Autodesk Inventor part; units mm, degrees
(part 2 of 2)
  spline S240 degree 2 poles (-24.576, 3.7543) (-24.576, 3.8655) (-24.644, 4.0034) (-24.7057, 4.0425) knots 0 0 0 1 2 2 2
  spline S241 degree 2 poles (-24.7057, 4.0425) (-24.7675, 4.0816) (-24.9445, 4.1063) (-25.0392, 4.1063) knots 0 0 0 1 2 2 2
  spline S242 degree 2 poles (-25.0392, 4.1063) (-25.1503, 4.1063) (-25.4508, 4.0404) (-25.6011, 3.9766) knots 0 0 0 1 2 2 2
  line L294 (-25.6011, 3.9766) -> (-25.6196, 3.9766)
  line L295 (-25.6196, 3.9766) -> (-25.6196, 4.3039)
  spline S243 degree 2 poles (-25.6196, 4.3039) (-25.5311, 4.3286) (-25.1997, 4.3903) (-25.0371, 4.3903) knots 0 0 0 1 2 2 2
  spline S244 degree 2 poles (-25.0371, 4.3903) (-24.8395, 4.3903) (-24.5699, 4.3286) (-24.4628, 4.2483) knots 0 0 0 1 2 2 2
  spline S245 degree 2 poles (-24.4628, 4.2483) (-24.3578, 4.1701) (-24.2549, 3.921) (-24.2549, 3.742) knots 0 0 0 1 2 2 2
  line L296 (-24.2549, 3.742) -> (-24.2549, 2.439)
  line L297 (-24.2549, 2.439) -> (-24.576, 2.439)
  line L298 (-24.576, 2.439) -> (-24.576, 2.6407)
  line L299 (-24.576, 2.9083) -> (-24.576, 3.4373)
  spline S246 degree 2 poles (-24.576, 3.4373) (-24.6913, 3.427) (-25.0392, 3.392) (-25.1482, 3.3591) knots 0 0 0 1 2 2 2
  spline S247 degree 2 poles (-25.1482, 3.3591) (-25.2759, 3.32) (-25.4426, 3.1574) (-25.4426, 3.0133) knots 0 0 0 1 2 2 2
  spline S248 degree 2 poles (-25.4426, 3.0133) (-25.4426, 2.8486) (-25.2573, 2.6819) (-25.0803, 2.6819) knots 0 0 0 1 2 2 2
  spline S249 degree 2 poles (-25.0803, 2.6819) (-24.9301, 2.6819) (-24.6831, 2.8116) (-24.576, 2.9083) knots 0 0 0 1 2 2 2
  line L300 (-20.836, 2.439) -> (-21.2744, 2.439)
  line L301 (-21.2744, 2.439) -> (-22.2028, 3.6205)
  line L302 (-22.2028, 3.6205) -> (-22.351, 3.4538)
  line L303 (-22.351, 3.4538) -> (-22.351, 2.439)
  line L304 (-22.351, 2.439) -> (-22.6885, 2.439)
  line L305 (-22.6885, 2.439) -> (-22.6885, 4.979)
  line L306 (-22.6885, 4.979) -> (-22.351, 4.979)
  line L307 (-22.351, 4.979) -> (-22.351, 3.8119)
  line L308 (-22.351, 3.8119) -> (-21.3094, 4.979)
  line L309 (-21.3094, 4.979) -> (-20.8978, 4.979)
  line L310 (-20.8978, 4.979) -> (-21.9496, 3.8449)
  line L311 (-21.9496, 3.8449) -> (-20.836, 2.439)
  line L312 (-19.6483, 4.0013) -> (-19.6648, 4.0013)
  spline S250 degree 2 poles (-19.6648, 4.0013) (-19.7019, 4.0116) (-19.7821, 4.0157) (-19.8377, 4.0157) knots 0 0 0 1 2 2 2
  spline S251 degree 2 poles (-19.8377, 4.0157) (-19.9674, 4.0157) (-20.2226, 3.9025) (-20.3379, 3.7914) knots 0 0 0 1 2 2 2
  line L313 (-20.3379, 3.7914) -> (-20.3379, 2.439)
  line L314 (-20.3379, 2.439) -> (-20.659, 2.439)
  line L315 (-20.659, 2.439) -> (-20.659, 4.3451)
  line L316 (-20.659, 4.3451) -> (-20.3379, 4.3451)
  line L317 (-20.3379, 4.3451) -> (-20.3379, 4.061)
  spline S252 degree 2 poles (-20.3379, 4.061) (-20.1629, 4.2174) (-19.9015, 4.3451) (-19.778, 4.3451) knots 0 0 0 1 2 2 2
  spline S253 degree 2 poles (-19.778, 4.3451) (-19.7286, 4.3451) (-19.6792, 4.3409) (-19.6483, 4.3348) knots 0 0 0 1 2 2 2
  line L318 (-19.6483, 4.3348) -> (-19.6483, 4.0013)
  line L319 (-19.6339, 5.2981) -> (-20.023, 4.6517)
  line L320 (-20.023, 4.6517) -> (-20.4099, 4.6517)
  line L321 (-20.4099, 4.6517) -> (-20.799, 5.2981)
  line L322 (-20.799, 5.2981) -> (-20.5273, 5.2981)
  line L323 (-20.5273, 5.2981) -> (-20.2123, 4.8617)
  line L324 (-20.2123, 4.8617) -> (-19.8974, 5.2981)
  line L325 (-19.8974, 5.2981) -> (-19.6339, 5.2981)
  line L326 (-19.072, 2.439) -> (-19.3931, 2.439)
  line L327 (-19.3931, 2.439) -> (-19.3931, 4.3451)
  line L328 (-19.3931, 4.3451) -> (-19.072, 4.3451)
  line L329 (-19.072, 4.3451) -> (-19.072, 2.439)
  line L330 (-19.0494, 4.662) -> (-19.4137, 4.662)
  line L331 (-19.4137, 4.662) -> (-19.4137, 4.9955)
  line L332 (-19.4137, 4.9955) -> (-19.0494, 4.9955)
  line L333 (-19.0494, 4.9955) -> (-19.0494, 4.662)
  line L334 (-17.3492, 2.439) -> (-18.7488, 2.439)
  line L335 (-18.7488, 2.439) -> (-18.7488, 2.6778)
  line L336 (-18.7488, 2.6778) -> (-17.7526, 4.0816)
  line L337 (-17.7526, 4.0816) -> (-18.7077, 4.0816)
  line L338 (-18.7077, 4.0816) -> (-18.7077, 4.3451)
  line L339 (-18.7077, 4.3451) -> (-17.3677, 4.3451)
  line L340 (-17.3677, 4.3451) -> (-17.3677, 4.1166)
  line L341 (-17.3677, 4.1166) -> (-18.3681, 2.7087)
  line L342 (-18.3681, 2.7087) -> (-17.3492, 2.7087)
  line L343 (-17.3492, 2.7087) -> (-17.3492, 2.439)
  line L344 (-17.4665, 5.2981) -> (-17.8555, 4.6517)
  line L345 (-17.8555, 4.6517) -> (-18.2425, 4.6517)
  line L346 (-18.2425, 4.6517) -> (-18.6315, 5.2981)
  line L347 (-18.6315, 5.2981) -> (-18.3598, 5.2981)
  line L348 (-18.3598, 5.2981) -> (-18.0449, 4.8617)
  line L349 (-18.0449, 4.8617) -> (-17.73, 5.2981)
  line L350 (-17.73, 5.2981) -> (-17.4665, 5.2981)
  line L351 (-16.7214, 2.439) -> (-17.0425, 2.439)
  line L352 (-17.0425, 2.439) -> (-17.0425, 4.3451)
  line L353 (-17.0425, 4.3451) -> (-16.7214, 4.3451)
  line L354 (-16.7214, 4.3451) -> (-16.7214, 2.439)
  line L355 (-16.355, 5.2981) -> (-16.8202, 4.66)
  line L356 (-16.8202, 4.66) -> (-17.0754, 4.66)
  line L357 (-17.0754, 4.66) -> (-16.7708, 5.2981)
  line L358 (-16.7708, 5.2981) -> (-16.355, 5.2981)
  line L359 (-14.6713, 2.439) -> (-15.0932, 2.439)
  line L360 (-15.0932, 2.439) -> (-15.8013, 3.3591)
  line L361 (-15.8013, 3.3591) -> (-15.9289, 3.2356)
  line L362 (-15.9289, 3.2356) -> (-15.9289, 2.439)
  line L363 (-15.9289, 2.439) -> (-16.25, 2.439)
  line L364 (-16.25, 2.439) -> (-16.25, 5.0922)
  line L365 (-16.25, 5.0922) -> (-15.9289, 5.0922)
  line L366 (-15.9289, 5.0922) -> (-15.9289, 3.5402)
  line L367 (-15.9289, 3.5402) -> (-15.1756, 4.3451)
  line L368 (-15.1756, 4.3451) -> (-14.7762, 4.3451)
  line L369 (-14.7762, 4.3451) -> (-15.5584, 3.5485)
  line L370 (-15.5584, 3.5485) -> (-14.6713, 2.439)
  spline S254 degree 2 poles (-13.4486, 2.6407) (-13.4877, 2.6119) (-13.6194, 2.509) (-13.6812, 2.4781) knots 0 0 0 1 2 2 2
  spline S255 degree 2 poles (-13.6812, 2.4781) (-13.7656, 2.4328) (-13.9241, 2.3855) (-14.0682, 2.3855) knots 0 0 0 1 2 2 2
  spline S256 degree 2 poles (-14.0682, 2.3855) (-14.1855, 2.3855) (-14.3975, 2.474) (-14.4778, 2.5543) knots 0 0 0 1 2 2 2
  spline S257 degree 2 poles (-14.4778, 2.5543) (-14.5539, 2.6325) (-14.6466, 2.863) (-14.6466, 2.9907) knots 0 0 0 1 2 2 2
  spline S258 degree 2 poles (-14.6466, 2.9907) (-14.6466, 3.1883) (-14.4798, 3.4682) (-14.2987, 3.5485) knots 0 0 0 1 2 2 2
  spline S259 degree 2 poles (-14.2987, 3.5485) (-14.1382, 3.6226) (-13.7018, 3.6781) (-13.4486, 3.6926) knots 0 0 0 1 2 2 2
  line L371 (-13.4486, 3.6926) -> (-13.4486, 3.7543)
  spline S260 degree 2 poles (-13.4486, 3.7543) (-13.4486, 3.8655) (-13.5165, 4.0034) (-13.5783, 4.0425) knots 0 0 0 1 2 2 2
  spline S261 degree 2 poles (-13.5783, 4.0425) (-13.64, 4.0816) (-13.817, 4.1063) (-13.9117, 4.1063) knots 0 0 0 1 2 2 2
  spline S262 degree 2 poles (-13.9117, 4.1063) (-14.0229, 4.1063) (-14.3234, 4.0404) (-14.4737, 3.9766) knots 0 0 0 1 2 2 2
  line L372 (-14.4737, 3.9766) -> (-14.4922, 3.9766)
  line L373 (-14.4922, 3.9766) -> (-14.4922, 4.3039)
  spline S263 degree 2 poles (-14.4922, 4.3039) (-14.4037, 4.3286) (-14.0723, 4.3903) (-13.9097, 4.3903) knots 0 0 0 1 2 2 2
  spline S264 degree 2 poles (-13.9097, 4.3903) (-13.7121, 4.3903) (-13.4424, 4.3286) (-13.3354, 4.2483) knots 0 0 0 1 2 2 2
  spline S265 degree 2 poles (-13.3354, 4.2483) (-13.2304, 4.1701) (-13.1275, 3.921) (-13.1275, 3.742) knots 0 0 0 1 2 2 2
  line L374 (-13.1275, 3.742) -> (-13.1275, 2.439)
  line L375 (-13.1275, 2.439) -> (-13.4486, 2.439)
  line L376 (-13.4486, 2.439) -> (-13.4486, 2.6407)
  line L377 (-13.4486, 2.9083) -> (-13.4486, 3.4373)
  spline S266 degree 2 poles (-13.4486, 3.4373) (-13.5639, 3.427) (-13.9117, 3.392) (-14.0208, 3.3591) knots 0 0 0 1 2 2 2
  spline S267 degree 2 poles (-14.0208, 3.3591) (-14.1484, 3.32) (-14.3152, 3.1574) (-14.3152, 3.0133) knots 0 0 0 1 2 2 2
  spline S268 degree 2 poles (-14.3152, 3.0133) (-14.3152, 2.8486) (-14.1299, 2.6819) (-13.9529, 2.6819) knots 0 0 0 1 2 2 2
  spline S269 degree 2 poles (-13.9529, 2.6819) (-13.8026, 2.6819) (-13.5556, 2.8116) (-13.4486, 2.9083) knots 0 0 0 1 2 2 2
  point P0 (0, -4.5)
  point P1 (-57.0087, 4.7786)
  point P2 (-54.5329, 8.3123)
  point P3 (-52.7402, 5.494)
  point P4 (-50.8019, 2.0843)
  point P5 (-46.9238, 7.9001)
  point P6 (-46.4946, 9)
  point P7 (-46.7114, 8.4844)
  constraints: 12 end point, 3 horizontal, 3 vertical, 2 point on line, 1 coincident, 18 other
sketch "Sketch5" plane through (48, 4.5, 0) normal (1, 0, 0) x (0, 0, -1)
  point P0 (0, -4.5)
extrude "Extrusion3" cut sketch "Sketch4" against normal blind 0.3
body "Solid1"
